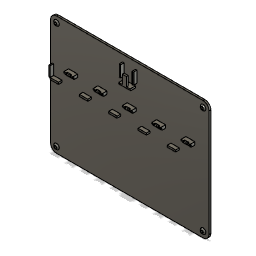
CP-BO Back v15 (Autodesk Fusion 360 design; units mm, degrees)
Autodesk Fusion 360 part; units mm, degrees
sketch "Esquisse1" plane through (0, 0, 0) normal (0, 0, 1) x (1, 0, 0)
  line L0 (10, 0) -> (255, 0)
  line L1 (265, 10) -> (265, 188.981)
  line L2 (255, 198.981) -> (10, 198.981)
  line L3 (0, 188.981) -> (0, 10)
  arc A0 (10, 198.981) -> (0, 188.981) centre (10, 188.981) ccw
  arc A1 (265, 188.981) -> (255, 198.981) centre (255, 188.981) ccw
  arc A2 (255, 0) -> (265, 10) centre (255, 10) ccw
  arc A3 (0, 10) -> (10, 0) centre (10, 10) ccw
  circle A4 centre (10, 188.981) radius 1.6
  circle A5 centre (255, 188.981) radius 1.6
  circle A6 centre (10, 10) radius 1.6
  circle A7 centre (255, 10) radius 1.6
  circle A8 centre (10, 188.981) radius 2.6
  circle A9 centre (10, 188.981) radius 3.5
  circle A10 centre (255, 188.981) radius 2.6
  circle A11 centre (255, 188.981) radius 3.5
  circle A12 centre (10, 10) radius 2.6
  circle A13 centre (10, 10) radius 3.5
  circle A14 centre (255, 10) radius 2.6
  circle A15 centre (255, 10) radius 3.5
  point P0 (265, 0)
  point P1 (0, 198.981)
  dimension "d1" = 265
  dimension "d2" = 198.981
  dimension "d3" = 10
  dimension "d6" = 3.2
  dimension "d9" = 245
  dimension "d10" = -178.981
  dimension "d13" = 5.2
  dimension "d14" = 7
  constraint horizontal L0
  constraint vertical L1
  constraint horizontal L2
  constraint vertical L3
  constraint coincident P1 L2
  constraint coincident P1 L3
  constraint tangent L2 A0
  constraint tangent L3 A0
  constraint tangent L1 A1
  constraint tangent L2 A1
  constraint equal A0 A1
  constraint coincident P0 L0
  constraint coincident P0 L1
  constraint tangent L0 A2
  constraint tangent L1 A2
  constraint equal A0 A2
  constraint coincident origin L0
  constraint coincident origin L3
  constraint tangent L0 A3
  constraint tangent L3 A3
  constraint equal A0 A3
  constraint concentric A0 A4
  constraint concentric A4 A8
  constraint concentric A0 A9
  measures "d1" distance of origin P0
  measures "d2" distance of origin P1
  measures "d3" radius of A0
  measures "d6" diameter of A4
  measures "d13" diameter of A8
  measures "d14" diameter of A9
extrude "trous de vis" add sketch "Esquisse1" along normal blind 3 contours L0 L1 L2 L3 A0 A1 A2 A3 | A8 | A9 | A10 | A11 | A12 | A13 | A14 | A15 makes body 1
extrude "Prolongation des trous" add sketch "Esquisse1" along normal blind 5 contours A8 | A10 | A12 | A14 bodies 1
extrude "Encastrement des vis" cut sketch "Esquisse1" along normal blind 2 contours A8 | A9 | A10 | A11 | A12 | A13 | A14 | A15 bodies 1
fillet "Renfort des prolongations des vis" radius 2 4 edges at (7.5759, 189.9212, 3) (7.5759, 10.9402, 3) (252.5759, 189.9212, 3) (252.5759, 10.9402, 3) on bodies 1
sketch "Support Arduino" plane through (0, 0, 3) normal (0, 0, 1) x (1, 0, 0)
  circle A0 centre (255, 188.981) radius 4.6
  circle A1 centre (10, 188.981) radius 4.6
  arc A2 (0, 10) -> (10, 0) centre (10, 10) ccw
  line L0 (10, 0) -> (255, 0)
  arc A3 (255, 0) -> (265, 10) centre (255, 10) ccw
  line L1 (265, 10) -> (265, 188.981)
  arc A4 (265, 188.981) -> (255, 198.981) centre (255, 188.981) ccw
  line L2 (255, 198.981) -> (10, 198.981)
  arc A5 (10, 198.981) -> (0, 188.981) centre (10, 188.981) ccw
  line L3 (0, 188.981) -> (0, 10)
  circle A6 centre (10, 10) radius 4.6
  circle A7 centre (255, 10) radius 4.6
  line L4 (132.5, 198.981) -> (132.5, 0) construction
  line L5 (76, 197.681) -> (188, 197.681) construction
  line L6 (255, 198.981) -> (10, 198.981) construction
  line L7 (123, 197.681) -> (142, 197.681) construction
  line L8 (142, 197.681) -> (142, 163.681) construction
  line L9 (142, 163.681) -> (123, 163.681) construction
  line L10 (123, 163.681) -> (123, 197.681) construction
  line L11 (123, 163.681) -> (142, 163.681)
  line L12 (142, 163.681) -> (142, 160.681)
  line L13 (142, 160.681) -> (123, 160.681)
  line L14 (123, 160.681) -> (123, 163.681)
  line L15 (142, 187.681) -> (144.5, 187.681)
  line L16 (144.5, 187.681) -> (144.5, 168.681)
  line L17 (144.5, 168.681) -> (142, 168.681)
  line L18 (142, 168.681) -> (142, 187.681)
  line L19 (123, 187.681) -> (120.5, 187.681)
  line L20 (120.5, 187.681) -> (120.5, 168.681)
  line L21 (120.5, 168.681) -> (123, 168.681)
  line L22 (123, 168.681) -> (123, 187.681)
  line L23 (120.5, 187.681) -> (152, 187.681) construction
  line L24 (120.5, 168.681) -> (153, 168.681) construction
  point P0 (10, 12.331)
  point P1 (255, 12.331)
  point P2 (10, 13.73)
  point P3 (255, 13.73)
  dimension "d21" = 1.3
  dimension "d22" = 19
  dimension "d23" = 34
  dimension "d24" = 2.5
  dimension "d25" = 2.5
  dimension "d27" = 5
  dimension "d28" = 10
  dimension "d29" = 3
  constraint midpoint L2 L4.start
  constraint midpoint L0 L4.end
  constraint parallel L5 L6
  constraint horizontal L7
  constraint vertical L8
  constraint horizontal L9
  constraint vertical L10
  constraint coincident L5 L7.start
  constraint symmetric L4 L8 L10
  constraint horizontal L11
  constraint vertical L12
  constraint horizontal L13
  constraint vertical L14
  constraint horizontal L15
  constraint vertical L16
  constraint horizontal L17
  constraint vertical L18
  constraint coincident L8 L15.start
  constraint horizontal L19
  constraint vertical L20
  constraint horizontal L21
  constraint vertical L22
  constraint coincident L10 L19.start
  constraint perpendicular L8 L23
  constraint coincident L15.end L23
  constraint perpendicular L8 L24
  constraint coincident L16.end L24
  measures "d21" distance of L5 L6
  measures "d22" distance of L8 L10
  measures "d23" distance of L5 L9
  measures "d24" distance of L20 L22
  measures "d25" distance of L8 L16
  measures "d27" distance of L11 L21
  measures "d28" distance of L5 L19
  measures "d29" distance of L11 L13
extrude "Cales latérales Arduino" add sketch "Support Arduino" along normal blind 6 contours L15 L16 L17 L18 | L19 L20 L21 L22 bodies 1
extrude "Cale arrière arduino" add sketch "Support Arduino" along normal blind 9 contours L11 L12 L13 L14 bodies 1
sketch "Sketch4" plane through (0, 163.681, 0) normal (0, 1, 0) x (-1, 0, 0)
  line L0 (-142, 3) -> (-123, 3)
  line L1 (-123, 3) -> (-123, 12)
  line L2 (-123, 12) -> (-142, 12)
  line L3 (-142, 12) -> (-142, 3)
  line L4 (-132.5, 3) -> (-132.5, 12) construction
  line L5 (-129, 12) -> (-136, 12)
  line L6 (-136, 12) -> (-136, 9)
  line L7 (-136, 9) -> (-129, 9)
  line L8 (-129, 9) -> (-129, 12)
  dimension "d34" = 7
  dimension "d35" = 3
  constraint midpoint L0 L4.start
  constraint midpoint L2 L4.end
  constraint horizontal L5
  constraint vertical L6
  constraint horizontal L7
  constraint vertical L8
  constraint coincident L2 L5.start
  constraint symmetric L4 L6 L8
  measures "d34" distance of L6 L8
  measures "d35" distance of L5 L7
extrude "Cale supérieure Arduino (1)" add sketch "Sketch4" along normal blind 15 contours L2 L5 L6 L7 L8 bodies 1
fillet "Fillet2" radius 1 3 edges at (120.5, 178.181, 9) (144.5, 178.181, 9) (132.5, 160.681, 12) on bodies 1
sketch "Esquisse2" plane through (0, 0, 3) normal (0, 0, 1) x (1, 0, 0)
  arc A0 (0, 10) -> (10, 0) centre (10, 10) ccw
  line L0 (10, 0) -> (255, 0)
  arc A1 (255, 0) -> (265, 10) centre (255, 10) ccw
  line L1 (265, 10) -> (265, 188.981)
  arc A2 (265, 188.981) -> (255, 198.981) centre (255, 188.981) ccw
  line L2 (255, 198.981) -> (10, 198.981)
  arc A3 (10, 198.981) -> (0, 188.981) centre (10, 188.981) ccw
  line L3 (0, 188.981) -> (0, 10)
  line L4 (0, 118.981) -> (265, 118.981) construction
  line L5 (5.2, 110.481) -> (5.2, 127.481) construction
  line L6 (5.2, 127.481) -> (249.2, 127.481) construction
  line L7 (249.2, 127.481) -> (249.2, 110.481) construction
  line L8 (249.2, 110.481) -> (5.2, 110.481) construction
  circle A4 centre (255, 188.981) radius 4.6
  circle A5 centre (10, 188.981) radius 4.6
  circle A6 centre (10, 10) radius 4.6
  circle A7 centre (255, 10) radius 4.6
  line L9 (123, 160.681) -> (123, 163.681)
  line L10 (123, 163.681) -> (142, 163.681)
  line L11 (142, 163.681) -> (142, 160.681)
  line L12 (142, 160.681) -> (123, 160.681)
  line L13 (142, 168.681) -> (142, 187.681)
  line L14 (142, 187.681) -> (144.5, 187.681)
  line L15 (144.5, 187.681) -> (144.5, 168.681)
  line L16 (144.5, 168.681) -> (142, 168.681)
  line L17 (123, 168.681) -> (120.5, 168.681)
  line L18 (120.5, 168.681) -> (120.5, 187.681)
  line L19 (120.5, 187.681) -> (123, 187.681)
  line L20 (123, 187.681) -> (123, 168.681)
  line L21 (3.2, 137.73) -> (3.2, 101.73) construction
  line L22 (3.2, 110.481) -> (5.2, 110.481)
  line L23 (5.2, 110.481) -> (5.2, 127.481)
  line L24 (5.2, 127.481) -> (3.2, 127.481)
  line L25 (3.2, 127.481) -> (3.2, 110.481)
  line L26 (5.2, 110.481) -> (19.2, 110.481)
  line L27 (19.2, 110.481) -> (19.2, 107.481)
  line L28 (19.2, 107.481) -> (5.2, 107.481)
  line L29 (5.2, 107.481) -> (5.2, 110.481)
  line L30 (54.2, 110.481) -> (68.2, 110.481)
  line L31 (68.2, 110.481) -> (68.2, 107.481)
  line L32 (68.2, 107.481) -> (54.2, 107.481)
  line L33 (54.2, 107.481) -> (54.2, 110.481)
  line L34 (103.2, 110.481) -> (117.2, 110.481)
  line L35 (117.2, 110.481) -> (117.2, 107.481)
  line L36 (117.2, 107.481) -> (103.2, 107.481)
  line L37 (103.2, 107.481) -> (103.2, 110.481)
  line L38 (152.2, 110.481) -> (166.2, 110.481)
  line L39 (166.2, 110.481) -> (166.2, 107.481)
  line L40 (166.2, 107.481) -> (152.2, 107.481)
  line L41 (152.2, 107.481) -> (152.2, 110.481)
  line L42 (230.0381, 107.481) -> (6.1619, 107.481) construction
  line L43 (201.2, 110.481) -> (215.2, 110.481)
  line L44 (215.2, 110.481) -> (215.2, 107.481)
  line L45 (215.2, 107.481) -> (201.2, 107.481)
  line L46 (201.2, 107.481) -> (201.2, 110.481)
  line L47 (249.2, 127.481) -> (257.2, 127.481) construction
  line L48 (257.2, 127.481) -> (257.2, 110.481) construction
  line L49 (257.2, 110.481) -> (249.2, 110.481) construction
  line L50 (249.2, 110.481) -> (249.2, 127.481) construction
  line L51 (3.0357, 132.481) -> (233.3856, 132.481) construction
  line L52 (30.2, 127.481) -> (45.2, 127.481)
  line L53 (45.2, 127.481) -> (45.2, 132.481)
  line L54 (45.2, 132.481) -> (30.2, 132.481)
  line L55 (30.2, 132.481) -> (30.2, 127.481)
  line L56 (30.2, 132.481) -> (34.2, 132.481)
  line L57 (34.2, 132.481) -> (34.2, 130.481)
  line L58 (34.2, 130.481) -> (30.2, 130.481)
  line L59 (30.2, 130.481) -> (30.2, 132.481)
  line L60 (45.2, 132.481) -> (41.2, 132.481)
  line L61 (41.2, 132.481) -> (41.2, 130.481)
  line L62 (41.2, 130.481) -> (45.2, 130.481)
  line L63 (45.2, 130.481) -> (45.2, 132.481)
  line L64 (79.2, 132.481) -> (94.2, 132.481)
  line L65 (94.2, 132.481) -> (94.2, 127.481)
  line L66 (94.2, 127.481) -> (79.2, 127.481)
  line L67 (79.2, 127.481) -> (79.2, 132.481)
  line L68 (128.2, 132.481) -> (143.2, 132.481)
  line L69 (143.2, 132.481) -> (143.2, 127.481)
  line L70 (143.2, 127.481) -> (128.2, 127.481)
  line L71 (128.2, 127.481) -> (128.2, 132.481)
  line L72 (177.2, 132.481) -> (192.2, 132.481)
  line L73 (192.2, 132.481) -> (192.2, 127.481)
  line L74 (192.2, 127.481) -> (177.2, 127.481)
  line L75 (177.2, 127.481) -> (177.2, 132.481)
  line L76 (226.2, 132.481) -> (241.2, 132.481)
  line L77 (241.2, 132.481) -> (241.2, 127.481)
  line L78 (241.2, 127.481) -> (226.2, 127.481)
  line L79 (226.2, 127.481) -> (226.2, 132.481)
  line L80 (1.8305, 130.481) -> (249.3342, 130.481) construction
  line L81 (79.2, 132.481) -> (83.2, 132.481)
  line L82 (83.2, 132.481) -> (83.2, 130.481)
  line L83 (83.2, 130.481) -> (79.2, 130.481)
  line L84 (79.2, 130.481) -> (79.2, 132.481)
  line L85 (94.2, 132.481) -> (90.2, 132.481)
  line L86 (90.2, 132.481) -> (90.2, 130.481)
  line L87 (90.2, 130.481) -> (94.2, 130.481)
  line L88 (94.2, 130.481) -> (94.2, 132.481)
  line L89 (128.2, 132.481) -> (132.2, 132.481)
  line L90 (132.2, 132.481) -> (132.2, 130.481)
  line L91 (132.2, 130.481) -> (128.2, 130.481)
  line L92 (128.2, 130.481) -> (128.2, 132.481)
  line L93 (143.2, 132.481) -> (139.2, 132.481)
  line L94 (139.2, 132.481) -> (139.2, 130.481)
  line L95 (139.2, 130.481) -> (143.2, 130.481)
  line L96 (143.2, 130.481) -> (143.2, 132.481)
  line L97 (177.2, 132.481) -> (181.2, 132.481)
  line L98 (181.2, 132.481) -> (181.2, 130.481)
  line L99 (181.2, 130.481) -> (177.2, 130.481)
  line L100 (177.2, 130.481) -> (177.2, 132.481)
  line L101 (192.2, 132.481) -> (188.2, 132.481)
  line L102 (188.2, 132.481) -> (188.2, 130.481)
  line L103 (188.2, 130.481) -> (192.2, 130.481)
  line L104 (192.2, 130.481) -> (192.2, 132.481)
  line L105 (226.2, 132.481) -> (230.2, 132.481)
  line L106 (230.2, 132.481) -> (230.2, 130.481)
  line L107 (230.2, 130.481) -> (226.2, 130.481)
  line L108 (226.2, 130.481) -> (226.2, 132.481)
  line L109 (241.2, 132.481) -> (237.2, 132.481)
  line L110 (237.2, 132.481) -> (237.2, 130.481)
  line L111 (237.2, 130.481) -> (241.2, 130.481)
  line L112 (241.2, 130.481) -> (241.2, 132.481)
  line L113 (37.7, 132.481) -> (37.7, 127.481) construction
  circle A8 centre (37.7, 129.981) radius 1.5
  line L114 (86.7, 132.481) -> (86.7, 127.481) construction
  line L115 (135.7, 132.481) -> (135.7, 127.481) construction
  line L116 (184.7, 132.481) -> (184.7, 127.481) construction
  line L117 (233.7, 132.481) -> (233.7, 127.481) construction
  circle A9 centre (86.7, 129.981) radius 1.5
  circle A10 centre (135.7, 129.981) radius 1.5
  circle A11 centre (184.7, 129.981) radius 1.5
  circle A12 centre (233.7, 129.981) radius 1.5
  point P0 (10, 12.331)
  point P1 (255, 12.331)
  point P2 (10, 13.73)
  point P3 (255, 13.73)
  dimension "d12" = 244
  dimension "d40" = 80
  dimension "d41" = 3.2
  dimension "d42" = 17
  dimension "d43" = 2
  dimension "d44" = 3
  dimension "d46" = 49
  dimension "d47" = 49
  dimension "d48" = 49
  dimension "d50" = 49
  dimension "d51" = 14
  dimension "d52" = 14
  dimension "d53" = 14
  dimension "d54" = 14
  dimension "d55" = 14
  dimension "d56" = 8
  dimension "d57" = 5
  dimension "d58" = 25
  dimension "d59" = 15
  dimension "d60" = 4
  dimension "d61" = 4
  dimension "d64" = 49
  dimension "d65" = 49
  dimension "d66" = 49
  dimension "d67" = 49
  dimension "d68" = 15
  dimension "d69" = 15
  dimension "d70" = 15
  dimension "d71" = 15
  dimension "d72" = 2
  dimension "d73" = 4
  dimension "d74" = 4
  dimension "d75" = 4
  dimension "d76" = 4
  dimension "d77" = 4
  dimension "d78" = 4
  dimension "d79" = 4
  dimension "d80" = 4
  dimension "d83" = 3
  dimension "d84" = 3
  dimension "d85" = 3
  dimension "d86" = 3
  dimension "d87" = 3
  constraint parallel L6 L8
  constraint parallel L4 L8
  constraint parallel L5 L7
  constraint perpendicular L5 L6
  constraint symmetric L4 L6 L8
  constraint parallel L2 L4
  constraint coincident L1 L4.end
  constraint coincident L3 L4.start
  constraint perpendicular L4 L21
  constraint horizontal L22
  constraint vertical L23
  constraint horizontal L24
  constraint vertical L25
  constraint coincident L21 L22.start
  constraint coincident L5.end L23
  constraint coincident L5.start L22
  constraint coincident L6 L5.end
  constraint horizontal L26
  constraint vertical L27
  constraint horizontal L28
  constraint vertical L29
  constraint coincident L8 L5.start
  constraint horizontal L30
  constraint vertical L31
  constraint horizontal L32
  constraint vertical L33
  constraint coincident L8 L30.start
  constraint horizontal L34
  constraint vertical L35
  constraint horizontal L36
  constraint vertical L37
  constraint horizontal L38
  constraint vertical L39
  constraint horizontal L40
  constraint vertical L41
  constraint coincident L8 L38.start
  constraint parallel L8 L42
  constraint coincident L39.end L42
  constraint coincident L35.end L42
  constraint coincident L27.end L42
  constraint coincident L31.end L42
  constraint horizontal L43
  constraint vertical L44
  constraint horizontal L45
  constraint vertical L46
  constraint coincident L42 L44.end
  constraint coincident L8 L43.start
  constraint coincident L5.start L8.end
  constraint horizontal L47
  constraint vertical L48
  constraint horizontal L49
  constraint vertical L50
  constraint coincident L7.end L8.start
  constraint parallel L6 L51
  constraint horizontal L52
  constraint vertical L53
  constraint horizontal L54
  constraint vertical L55
  constraint coincident L51 L53.end
  constraint coincident L6 L52.start
  constraint horizontal L56
  constraint vertical L57
  constraint horizontal L58
  constraint vertical L59
  constraint horizontal L60
  constraint vertical L61
  constraint horizontal L62
  constraint vertical L63
  constraint horizontal L64
  constraint vertical L65
  constraint horizontal L66
  constraint vertical L67
  constraint coincident L6 L65.end
  constraint coincident L51 L64.start
  constraint horizontal L68
  constraint vertical L69
  constraint horizontal L70
  constraint vertical L71
  constraint coincident L6 L69.end
  constraint coincident L51 L68.start
  constraint horizontal L72
  constraint vertical L73
  constraint horizontal L74
  constraint vertical L75
  constraint coincident L6 L73.end
  constraint coincident L51 L72.start
  constraint horizontal L76
  constraint vertical L77
  constraint horizontal L78
  constraint vertical L79
  constraint coincident L6 L77.end
  constraint coincident L51 L76.start
  constraint parallel L51 L80
  constraint coincident L57.end L80
  constraint coincident L62.end L80
  constraint horizontal L81
  constraint vertical L82
  constraint horizontal L83
  constraint vertical L84
  constraint horizontal L85
  constraint vertical L86
  constraint horizontal L87
  constraint vertical L88
  constraint horizontal L89
  constraint vertical L90
  constraint horizontal L91
  constraint vertical L92
  constraint horizontal L93
  constraint vertical L94
  constraint horizontal L95
  constraint vertical L96
  constraint horizontal L97
  constraint vertical L98
  constraint horizontal L99
  constraint vertical L100
  constraint horizontal L101
  constraint vertical L102
  constraint horizontal L103
  constraint vertical L104
  constraint horizontal L105
  constraint vertical L106
  constraint horizontal L107
  constraint vertical L108
  constraint horizontal L109
  constraint vertical L110
  constraint horizontal L111
  constraint vertical L112
  constraint midpoint L54 L113.start
  constraint midpoint L52 L113.end
  constraint midpoint L113 A8.centre
  constraint midpoint L64 L114.start
  constraint midpoint L66 L114.end
  constraint midpoint L68 L115.start
  constraint midpoint L70 L115.end
  constraint midpoint L72 L116.start
  constraint midpoint L74 L116.end
  constraint midpoint L76 L117.start
  constraint midpoint L78 L117.end
  constraint midpoint L114 A9.centre
  constraint midpoint L115 A10.centre
  constraint midpoint L116 A11.centre
  constraint midpoint L117 A12.centre
  constraint coincident L80 L82.end
  constraint coincident L80 L86.end
  constraint coincident L80 L90.end
  constraint coincident L80 L94.end
  constraint coincident L80 L98.end
  constraint coincident L80 L102.end
  constraint coincident L80 L106.end
  constraint coincident L80 L110.end
  measures "d12" distance of L5 L7
  measures "d40" distance of L2 L4
  measures "d41" distance of L3 L21
  measures "d42" distance of L22 L24
  measures "d43" distance of L23 L25
  measures "d44" distance of L8 L42
  measures "d46" distance of L29 L33
  measures "d47" distance of L33 L37
  measures "d48" distance of L37 L41
  measures "d50" distance of L41 L46
  measures "d51" distance of L27 L29
  measures "d52" distance of L31 L33
  measures "d53" distance of L35 L37
  measures "d54" distance of L39 L41
  measures "d55" distance of L44 L46
  measures "d56" distance of L7 L48
  measures "d57" distance of L47 L51
  measures "d58" distance of L5.end L55
  measures "d59" distance of L53 L55
  measures "d60" distance of L54.end L56.end
  measures "d61" distance of L53.end L60.end
  measures "d64" distance of L55 L67
  measures "d65" distance of L67 L71
  measures "d66" distance of L71 L75
  measures "d67" distance of L75 L79
  measures "d68" distance of L65 L67
  measures "d69" distance of L69 L71
  measures "d70" distance of L73 L75
  measures "d71" distance of L77 L79
  measures "d72" distance of L51 L80
  measures "d73" distance of L64.start L81.end
  measures "d74" distance of L64.end L85.end
  measures "d75" distance of L68.start L89.end
  measures "d76" distance of L68.end L93.end
  measures "d77" distance of L72.start L97.end
  measures "d78" distance of L72.end L101.end
  measures "d79" distance of L76.start L105.end
  measures "d80" distance of L76.end L109.end
  measures "d83" diameter of A8
  measures "d84" diameter of A9
  measures "d85" diameter of A10
  measures "d86" diameter of A11
  measures "d87" diameter of A12
extrude "Cales PCF" add sketch "Esquisse2" along normal blind 6 separate body contours L22 L23 L24 L25 | L26 L27 L28 L29 | L30 L31 L32 L33 | L34 L35 L36 L37 | L38 L39 L40 L41 | L43 L44 L45 L46 | L52 L53 L54 L55 L57 L58 L61 L62 | L64 L65 L66 L67 L82 L83 L86 L87 | L68 L69 L70 L71 L90 L91 L94 L95 | L72 L73 L74 L75 L98 L99 L102 L103 | L76 L77 L78 L79 L106 L107 L110 L111 makes body 8 at (3.2, 121.8143, 5) makes body 8 at (9.8667, 110.481, 5) makes body 9 at (58.8667, 110.481, 5) makes body 4 at (107.8667, 110.481, 5) makes body 3 at (156.8667, 110.481, 5) makes body 7 at (210.5333, 107.481, 5) makes body 2 at (35.2, 127.481, 5) makes body 6 at (89.2, 127.481, 7) makes body 11 at (138.2, 127.481, 7) makes body 5 at (187.2, 127.481, 7) makes body 10 at (236.2, 127.481, 7)
extrude "Cales pour supports" add sketch "Esquisse2" along normal blind 8 contours L54 L55 L56 L57 L58 L59 | L53 L54 L60 L61 L62 L63 | L64 L67 L81 L82 L83 L84 | L64 L65 L85 L86 L87 L88 | L68 L71 L89 L90 L91 L92 | L68 L69 L93 L94 L95 L96 | L72 L75 L97 L98 L99 L100 | L72 L73 L101 L102 L103 L104 | L76 L79 L105 L106 L107 L108 | L76 L77 L109 L110 L111 L112 bodies 1 2 5 6 10 11
